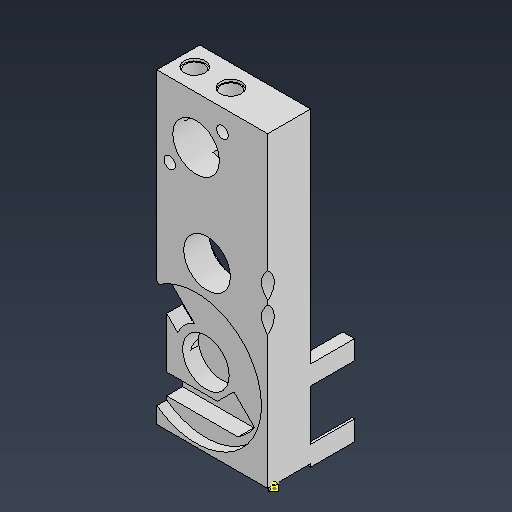
# Autodesk Inventor part: Left_gearbox
Saved by Autodesk Inventor 2026.2 (Build 302298010, 298A)
## iProperties
Created: 2026-04-03
Part Number: Left_gearbox
Material: Generic
Document SubType Name: Modeling
Designer: szymo
Density: 1 g/cm^3
Appearance: Default
Mass: 8.18734 g
Surface Area: 67.5821 cm^2
Volume: 8.18734 cm^3
Author: szymo
Autodesk Inventor part; units mm, degrees
(part 1 of 2)
ref_plane "YZ Plane" through (0, 0, 0) normal (1, 0, 0) x (0, 1, 0)
ref_plane "XZ Plane" through (0, 0, 0) normal (0, 1, 0) x (-1, 0, 0)
ref_plane "XY Plane" through (0, 0, 0) normal (0, 0, 1) x (1, 0, 0)
sketch "Sketch2" plane through (0, 0, 0) normal (0, 0, 1) x (1, 0, 0)
  circle A0 centre (-9.6931, 61.9439) radius 1.0564 construction
  circle A1 centre (-21.0069, 50.6302) radius 1.0564 construction
  circle A2 centre (-15.35, 56.2871) radius 5 projected
  circle A3 centre (-15.35, 56.2871) radius 14 construction
  circle A4 centre (-9.652, 48.0693) radius 1.25 construction
  arc A5 (-9.9568, 54.9375) -> (-10.4245, 56.0319) centre (-14.7581, 53.5328) ccw construction
  arc A6 (-9.5969, 54.944) -> (-9.9568, 54.9375) centre (-9.652, 48.0693) ccw construction
  arc A7 (-9.1694, 56.0547) -> (-9.5969, 54.944) centre (-4.7478, 53.7148) ccw construction
  arc A8 (-8.7521, 56.0185) -> (-9.1694, 56.0547) centre (-9.652, 48.0693) ccw construction
  arc A9 (-8.5222, 54.8508) -> (-8.7521, 56.0185) centre (-13.5106, 54.4751) ccw construction
  arc A10 (-8.1688, 54.7824) -> (-8.5222, 54.8508) centre (-9.652, 48.0693) ccw construction
  arc A11 (-7.5196, 55.7798) -> (-8.1688, 54.7824) centre (-3.6812, 52.5718) ccw construction
  arc A12 (-7.119, 55.6577) -> (-7.5196, 55.7798) centre (-9.652, 48.0693) ccw construction
  arc A13 (-7.1369, 54.4677) -> (-7.119, 55.6577) centre (-12.0944, 55.1373) ccw construction
  arc A14 (-6.8055, 54.3273) -> (-7.1369, 54.4677) centre (-9.652, 48.0693) ccw construction
  arc A15 (-5.9631, 55.168) -> (-6.8055, 54.3273) centre (-2.8755, 51.232) ccw construction
  arc A16 (-5.5966, 54.9652) -> (-5.9631, 55.168) centre (-9.652, 48.0693) ccw construction
  arc A17 (-5.8615, 53.805) -> (-5.5966, 54.9652) centre (-10.5715, 55.4907) ccw construction
  arc A18 (-5.5666, 53.5987) -> (-5.8615, 53.805) centre (-9.652, 48.0693) ccw construction
  arc A19 (-4.5678, 54.2459) -> (-5.5666, 53.5987) centre (-2.366, 49.754) ccw construction
  arc A20 (-4.2515, 53.9714) -> (-4.5678, 54.2459) centre (-9.652, 48.0693) ccw construction
  arc A21 (-4.7519, 52.8916) -> (-4.2515, 53.9714) centre (-9.0084, 55.5197) ccw construction
  arc A22 (-4.5062, 52.6285) -> (-4.7519, 52.8916) centre (-9.652, 48.0693) ccw construction
  arc A23 (-3.3947, 53.0539) -> (-4.5062, 52.6285) centre (-2.175, 48.2023) ccw construction
  arc A24 (-3.1424, 52.7196) -> (-3.3947, 53.0539) centre (-9.652, 48.0693) ccw construction
  arc A25 (-3.8563, 51.7674) -> (-3.1424, 52.7196) centre (-7.4735, 55.2231) ccw construction
  arc A26 (-3.6707, 51.459) -> (-3.8563, 51.7674) centre (-9.652, 48.0693) ccw construction
  arc A27 (-2.4951, 51.644) -> (-3.6707, 51.459) centre (-2.3107, 46.6449) ccw construction
  arc A28 (-2.3178, 51.2646) -> (-2.4951, 51.644) centre (-9.652, 48.0693) ccw construction
  arc A29 (-3.2141, 50.4816) -> (-2.3178, 51.2646) centre (-6.0337, 54.6138) ccw construction
  arc A30 (-3.0967, 50.1413) -> (-3.2141, 50.4816) centre (-9.652, 48.0693) ccw construction
  arc A31 (-1.9082, 50.0779) -> (-3.0967, 50.1413) centre (-2.7673, 45.1497) ccw construction
  arc A32 (-1.8137, 49.6699) -> (-1.9082, 50.0779) centre (-9.652, 48.0693) ccw construction
  arc A33 (-2.8532, 49.0904) -> (-1.8137, 49.6699) centre (-4.7521, 53.7185) ccw construction
  arc A34 (-2.8091, 48.7331) -> (-2.8532, 49.0904) centre (-9.652, 48.0693) ccw construction
  arc A35 (-1.6598, 48.424) -> (-2.8091, 48.7331) centre (-3.5247, 43.7821) ccw construction
  arc A36 (-1.6522, 48.0052) -> (-1.6598, 48.424) centre (-9.652, 48.0693) ccw construction
  arc A37 (-2.7895, 47.6545) -> (-1.6522, 48.0052) centre (-3.6846, 52.5763) ccw construction
  arc A38 (-2.8206, 47.2959) -> (-2.7895, 47.6545) centre (-9.652, 48.0693) ccw construction
  arc A39 (-1.7607, 46.7546) -> (-2.8206, 47.2959) centre (-4.55, 42.6018) ccw construction
  arc A40 (-1.8404, 46.3434) -> (-1.7607, 46.7546) centre (-9.652, 48.0693) ccw construction
  arc A41 (-3.0257, 46.2368) -> (-1.8404, 46.3434) centre (-2.8779, 51.2371) ccw construction
  arc A42 (-3.1307, 45.8925) -> (-3.0257, 46.2368) centre (-9.652, 48.0693) ccw construction
  arc A43 (-2.2065, 45.1426) -> (-3.1307, 45.8925) centre (-5.7982, 41.6605) ccw construction
  arc A44 (-2.3699, 44.757) -> (-2.2065, 45.1426) centre (-9.652, 48.0693) ccw construction
  arc A45 (-3.5515, 44.8991) -> (-2.3699, 44.757) centre (-2.3673, 49.7595) ccw construction
  arc A46 (-3.7258, 44.5842) -> (-3.5515, 44.8991) centre (-9.652, 48.0693) ccw construction
  arc A47 (-2.9777, 43.6586) -> (-3.7258, 44.5842) centre (-7.2149, 40.9993) ccw construction
  arc A48 (-3.2177, 43.3153) -> (-2.9777, 43.6586) centre (-9.652, 48.0693) ccw construction
  arc A49 (-4.3439, 43.7001) -> (-3.2177, 43.3153) centre (-2.1751, 48.208) ccw construction
  arc A50 (-4.5798, 43.4282) -> (-4.3439, 43.7001) centre (-9.652, 48.0693) ccw construction
  arc A51 (-4.0406, 42.3673) -> (-4.5798, 43.4282) centre (-8.7381, 40.6471) ccw construction
  arc A52 (-4.3467, 42.0814) -> (-4.0406, 42.3673) centre (-9.652, 48.0693) ccw construction
  arc A53 (-5.3683, 42.6919) -> (-4.3467, 42.0814) centre (-2.3096, 46.6504) ccw construction
  arc A54 (-5.6556, 42.4751) -> (-5.3683, 42.6919) centre (-9.652, 48.0693) ccw construction
  arc A55 (-5.3487, 41.3252) -> (-5.6556, 42.4751) centre (-10.3012, 40.6193) ccw construction
  arc A56 (-5.7076, 41.1093) -> (-5.3487, 41.3252) centre (-9.652, 48.0693) ccw construction
  arc A57 (-6.5799, 41.9188) -> (-5.7076, 41.1093) centre (-2.7651, 45.1549) ccw construction
  arc A58 (-6.906, 41.7665) -> (-6.5799, 41.9188) centre (-9.652, 48.0693) ccw construction
  arc A59 (-6.8449, 40.5779) -> (-6.906, 41.7665) centre (-11.8359, 40.9171) ccw construction
  arc A60 (-7.2408, 40.4413) -> (-6.8449, 40.5779) centre (-9.652, 48.0693) ccw construction
  arc A61 (-7.9258, 41.4145) -> (-7.2408, 40.4413) centre (-3.5215, 43.7867) ccw construction
  arc A62 (-8.2764, 41.3333) -> (-7.9258, 41.4145) centre (-9.652, 48.0693) ccw construction
  arc A63 (-8.4638, 40.158) -> (-8.2764, 41.3333) centre (-13.2752, 41.5275) ccw construction
  arc A64 (-8.8795, 40.1066) -> (-8.4638, 40.158) centre (-9.652, 48.0693) ccw construction
  arc A65 (-9.3471, 41.201) -> (-8.8795, 40.1066) centre (-4.5458, 42.6057) ccw construction
  arc A66 (-9.707, 41.1945) -> (-9.3471, 41.201) centre (-9.652, 48.0693) ccw construction
  arc A67 (-10.1346, 40.0838) -> (-9.707, 41.1945) centre (-14.5562, 42.4237) ccw construction
  arc A68 (-10.5519, 40.12) -> (-10.1346, 40.0838) centre (-9.652, 48.0693) ccw construction
  arc A69 (-10.7818, 41.2877) -> (-10.5519, 40.12) centre (-5.7934, 41.6635) ccw construction
  arc A70 (-11.1351, 41.3561) -> (-10.7818, 41.2877) centre (-9.652, 48.0693) ccw construction
  arc A71 (-11.7843, 40.3587) -> (-11.1351, 41.3561) centre (-15.6228, 43.5667) ccw construction
  arc A72 (-12.1849, 40.4808) -> (-11.7843, 40.3587) centre (-9.652, 48.0693) ccw construction
  arc A73 (-12.167, 41.6708) -> (-12.1849, 40.4808) centre (-7.2095, 41.0012) ccw construction
  arc A74 (-12.4985, 41.8112) -> (-12.167, 41.6708) centre (-9.652, 48.0693) ccw construction
  arc A75 (-13.3408, 40.9705) -> (-12.4985, 41.8112) centre (-16.4284, 44.9065) ccw construction
  arc A76 (-13.7073, 41.1733) -> (-13.3408, 40.9705) centre (-9.652, 48.0693) ccw construction
  arc A77 (-13.4424, 42.3336) -> (-13.7073, 41.1733) centre (-8.7324, 40.6478) ccw construction
  arc A78 (-13.7374, 42.5398) -> (-13.4424, 42.3336) centre (-9.652, 48.0693) ccw construction
  arc A79 (-14.7361, 41.8926) -> (-13.7374, 42.5398) centre (-16.9379, 46.3845) ccw construction
  arc A80 (-15.0524, 42.1671) -> (-14.7361, 41.8926) centre (-9.652, 48.0693) ccw construction
  arc A81 (-14.5521, 43.247) -> (-15.0524, 42.1671) centre (-10.2955, 40.6188) ccw construction
  arc A82 (-14.7977, 43.51) -> (-14.5521, 43.247) centre (-9.652, 48.0693) ccw construction
  arc A83 (-15.9092, 43.0846) -> (-14.7977, 43.51) centre (-17.129, 47.9362) ccw construction
  arc A84 (-16.1615, 43.4189) -> (-15.9092, 43.0846) centre (-9.652, 48.0693) ccw construction
  arc A85 (-15.4476, 44.3711) -> (-16.1615, 43.4189) centre (-11.8305, 40.9154) ccw construction
  arc A86 (-15.6332, 44.6795) -> (-15.4476, 44.3711) centre (-9.652, 48.0693) ccw construction
  arc A87 (-16.8089, 44.4945) -> (-15.6332, 44.6795) centre (-16.9932, 49.4936) ccw construction
  arc A88 (-16.9861, 44.874) -> (-16.8089, 44.4945) centre (-9.652, 48.0693) ccw construction
  arc A89 (-16.0899, 45.6569) -> (-16.9861, 44.874) centre (-13.2702, 41.5247) ccw construction
  arc A90 (-16.2073, 45.9972) -> (-16.0899, 45.6569) centre (-9.652, 48.0693) ccw construction
  arc A91 (-17.3957, 46.0606) -> (-16.2073, 45.9972) centre (-16.5367, 50.9889) ccw construction
  arc A92 (-17.4902, 46.4687) -> (-17.3957, 46.0606) centre (-9.652, 48.0693) ccw construction
  arc A93 (-16.4507, 47.0482) -> (-17.4902, 46.4687) centre (-14.5519, 42.42) ccw construction
  arc A94 (-16.4948, 47.4054) -> (-16.4507, 47.0482) centre (-9.652, 48.0693) ccw construction
  arc A95 (-17.6441, 47.7145) -> (-16.4948, 47.4054) centre (-15.7792, 52.3565) ccw construction
  arc A96 (-17.6517, 48.1333) -> (-17.6441, 47.7145) centre (-9.652, 48.0693) ccw construction
  arc A97 (-16.5144, 48.484) -> (-17.6517, 48.1333) centre (-15.6193, 43.5622) ccw construction
  arc A98 (-16.4833, 48.8426) -> (-16.5144, 48.484) centre (-9.652, 48.0693) ccw construction
  arc A99 (-17.5432, 49.3839) -> (-16.4833, 48.8426) centre (-14.7539, 53.5367) ccw construction
  arc A100 (-17.4636, 49.7951) -> (-17.5432, 49.3839) centre (-9.652, 48.0693) ccw construction
  arc A101 (-16.2783, 49.9017) -> (-17.4636, 49.7951) centre (-16.426, 44.9014) ccw construction
  arc A102 (-16.1733, 50.246) -> (-16.2783, 49.9017) centre (-9.652, 48.0693) ccw construction
  arc A103 (-17.0974, 50.9959) -> (-16.1733, 50.246) centre (-13.5057, 54.478) ccw construction
  arc A104 (-16.9341, 51.3815) -> (-17.0974, 50.9959) centre (-9.652, 48.0693) ccw construction
  arc A105 (-15.7525, 51.2394) -> (-16.9341, 51.3815) centre (-16.9366, 46.379) ccw construction
  arc A106 (-15.5782, 51.5543) -> (-15.7525, 51.2394) centre (-9.652, 48.0693) ccw construction
  arc A107 (-16.3262, 52.4799) -> (-15.5782, 51.5543) centre (-12.089, 55.1392) ccw construction
  arc A108 (-16.0863, 52.8232) -> (-16.3262, 52.4799) centre (-9.652, 48.0693) ccw construction
  arc A109 (-14.96, 52.4385) -> (-16.0863, 52.8232) centre (-17.1289, 47.9305) ccw construction
  arc A110 (-14.7241, 52.7103) -> (-14.96, 52.4385) centre (-9.652, 48.0693) ccw construction
  arc A111 (-15.2634, 53.7712) -> (-14.7241, 52.7103) centre (-10.5659, 55.4914) ccw construction
  arc A112 (-14.9573, 54.0571) -> (-15.2634, 53.7712) centre (-9.652, 48.0693) ccw construction
  arc A113 (-13.9356, 53.4466) -> (-14.9573, 54.0571) centre (-16.9943, 49.4881) ccw construction
  arc A114 (-13.6483, 53.6634) -> (-13.9356, 53.4466) centre (-9.652, 48.0693) ccw construction
  arc A115 (-13.9552, 54.8133) -> (-13.6483, 53.6634) centre (-9.0028, 55.5192) ccw construction
  arc A116 (-13.5964, 55.0293) -> (-13.9552, 54.8133) centre (-9.652, 48.0693) ccw construction
  arc A117 (-12.724, 54.2197) -> (-13.5964, 55.0293) centre (-16.5389, 50.9836) ccw construction
  arc A118 (-12.3979, 54.3721) -> (-12.724, 54.2197) centre (-9.652, 48.0693) ccw construction
  arc A119 (-12.459, 55.5606) -> (-12.3979, 54.3721) centre (-7.468, 55.2214) ccw construction
  arc A120 (-12.0631, 55.6973) -> (-12.459, 55.5606) centre (-9.652, 48.0693) ccw construction
  arc A121 (-11.3781, 54.724) -> (-12.0631, 55.6973) centre (-15.7825, 52.3518) ccw construction
  arc A122 (-11.0275, 54.8052) -> (-11.3781, 54.724) centre (-9.652, 48.0693) ccw construction
  arc A123 (-10.8402, 55.9805) -> (-11.0275, 54.8052) centre (-6.0287, 54.6111) ccw construction
  arc A124 (-10.4245, 56.0319) -> (-10.8402, 55.9805) centre (-9.652, 48.0693) ccw construction
  circle A125 centre (-13, 35.9222) radius 5 projected
  arc A126 (-10.4838, 26.6578) -> (-10.4239, 28.0847) centre (-16.409, 27.6212) ccw construction
  arc A127 (-10.4239, 28.0847) -> (-10.0173, 28.2303) centre (-13, 35.9222) ccw construction
  arc A128 (-10.0173, 28.2303) -> (-9.0655, 27.1655) centre (-5.0975, 31.6701) ccw construction
  arc A129 (-9.0655, 27.1655) -> (-8.6126, 27.3834) centre (-13, 35.9222) ccw construction
  arc A130 (-8.6126, 27.3834) -> (-8.8507, 28.7916) centre (-14.6087, 27.0938) ccw construction
  arc A131 (-8.8507, 28.7916) -> (-8.4832, 29.0185) centre (-13, 35.9222) ccw construction
  arc A132 (-8.4832, 29.0185) -> (-7.3309, 28.1749) centre (-4.3862, 33.4061) ccw construction
  arc A133 (-7.3309, 28.1749) -> (-6.9332, 28.4822) centre (-13, 35.9222) ccw construction
  arc A134 (-6.9332, 28.4822) -> (-7.4588, 29.8101) centre (-12.738, 26.9522) ccw construction
  arc A135 (-7.4588, 29.8101) -> (-7.1466, 30.1085) centre (-13, 35.9222) ccw construction
  arc A136 (-7.1466, 30.1085) -> (-5.844, 29.5229) centre (-4.0513, 35.252) ccw construction
  arc A137 (-5.844, 29.5229) -> (-5.5189, 29.9062) centre (-13, 35.9222) ccw construction
  arc A138 (-5.5189, 29.9062) -> (-6.3091, 31.0957) centre (-10.8787, 27.2027) ccw construction
  arc A139 (-6.3091, 31.0957) -> (-6.0657, 31.4525) centre (-13, 35.9222) ccw construction
  arc A140 (-6.0657, 31.4525) -> (-4.6699, 31.1505) centre (-4.1075, 37.1272) ccw construction
  arc A141 (-4.6699, 31.1505) -> (-4.4316, 31.593) centre (-13, 35.9222) ccw construction
  arc A142 (-4.4316, 31.593) -> (-5.4519, 32.5923) centre (-9.1122, 27.8343) ccw construction
  arc A143 (-5.4519, 32.5923) -> (-5.2879, 32.9919) centre (-13, 35.9222) ccw construction
  arc A144 (-5.2879, 32.9919) -> (-3.8598, 32.9867) centre (-4.5523, 38.9497) ccw construction
  arc A145 (-3.8598, 32.9867) -> (-3.7187, 33.4691) centre (-13, 35.9222) ccw construction
  arc A146 (-3.7187, 33.4691) -> (-4.9245, 34.2344) centre (-7.5156, 28.8194) ccw construction
  arc A147 (-4.9245, 34.2344) -> (-4.8472, 34.6594) centre (-13, 35.9222) ccw construction
  arc A148 (-4.8472, 34.6594) -> (-3.4492, 34.9512) centre (-5.3664, 40.6399) ccw construction
  arc A149 (-3.4492, 34.9512) -> (-3.4115, 35.4524) centre (-13, 35.9222) ccw construction
  arc A150 (-3.4115, 35.4524) -> (-4.75, 35.9503) centre (-6.1587, 30.1148) ccw construction
  arc A151 (-4.75, 35.9503) -> (-4.7628, 36.382) centre (-13, 35.9222) ccw construction
  arc A152 (-4.7628, 36.382) -> (-3.4561, 36.9582) centre (-6.514, 42.124) ccw construction
  arc A153 (-3.4561, 36.9582) -> (-3.5234, 37.4562) centre (-13, 35.9222) ccw construction
  arc A154 (-3.5234, 37.4562) -> (-4.9362, 37.6649) centre (-5.1008, 31.6641) ccw construction
  arc A155 (-4.9362, 37.6649) -> (-5.0384, 38.0846) centre (-13, 35.9222) ccw construction
  arc A156 (-5.0384, 38.0846) -> (-3.88, 38.9198) centre (-7.9452, 43.3369) ccw construction
  arc A157 (-3.88, 38.9198) -> (-4.0494, 39.393) centre (-13, 35.9222) ccw construction
  arc A158 (-4.0494, 39.393) -> (-5.4747, 39.3034) centre (-4.3881, 33.3995) ccw construction
  arc A159 (-5.4747, 39.3034) -> (-5.662, 39.6926) centre (-13, 35.9222) ccw construction
  arc A160 (-5.662, 39.6926) -> (-4.7025, 40.7505) centre (-9.5973, 44.2259) ccw construction
  arc A161 (-4.7025, 40.7505) -> (-4.9666, 41.1781) centre (-13, 35.9222) ccw construction
  arc A162 (-4.9666, 41.1781) -> (-6.3422, 40.7941) centre (-4.0518, 35.2452) ccw construction
  arc A163 (-6.3422, 40.7941) -> (-6.6063, 41.1359) centre (-13, 35.9222) ccw construction
  arc A164 (-6.6063, 41.1359) -> (-5.8877, 42.3701) centre (-11.398, 44.7519) ccw construction
  arc A165 (-5.8877, 42.3701) -> (-6.2349, 42.7335) centre (-13, 35.9222) ccw construction
  arc A166 (-6.2349, 42.7335) -> (-7.5006, 42.0719) centre (-4.1066, 37.1204) ccw construction
  arc A167 (-7.5006, 42.0719) -> (-7.83, 42.3513) centre (-13, 35.9222) ccw construction
  arc A168 (-7.83, 42.3513) -> (-7.3837, 43.7079) centre (-13.2688, 44.892) ccw construction
  arc A169 (-7.3837, 43.7079) -> (-7.7989, 43.9912) centre (-13, 35.9222) ccw construction
  arc A170 (-7.7989, 43.9912) -> (-8.8993, 43.0809) centre (-4.55, 38.9433) ccw construction
  arc A171 (-8.8993, 43.0809) -> (-9.2796, 43.2857) centre (-13, 35.9222) ccw construction
  arc A172 (-9.2796, 43.2857) -> (-9.1252, 44.7055) centre (-15.1279, 44.6401) ccw construction
  arc A173 (-9.1252, 44.7055) -> (-9.5902, 44.8962) centre (-13, 35.9222) ccw construction
  arc A174 (-9.5902, 44.8962) -> (-10.4773, 43.7771) centre (-5.3628, 40.6341) ccw construction
  arc A175 (-10.4773, 43.7771) -> (-10.8919, 43.8983) centre (-13, 35.9222) ccw construction
  arc A176 (-10.8919, 43.8983) -> (-11.036, 45.3192) centre (-16.8939, 44.0072) ccw construction
  arc A177 (-11.036, 45.3192) -> (-11.5305, 45.4091) centre (-13, 35.9222) ccw construction
  arc A178 (-11.5305, 45.4091) -> (-12.1656, 44.1299) centre (-6.5093, 42.119) ccw construction
  arc A179 (-12.1656, 44.1299) -> (-12.5963, 44.1623) centre (-13, 35.9222) ccw construction
  arc A180 (-12.5963, 44.1623) -> (-13.0327, 45.5222) centre (-18.4898, 43.0209) ccw construction
  arc A181 (-13.0327, 45.5222) -> (-13.535, 45.5073) centre (-13, 35.9222) ccw construction
  arc A182 (-13.535, 45.5073) -> (-13.8903, 44.124) centre (-7.9396, 43.3331) ccw construction
  arc A183 (-13.8903, 44.124) -> (-14.3183, 44.0662) centre (-13, 35.9222) ccw construction
  arc A184 (-14.3183, 44.0662) -> (-15.0279, 45.3056) centre (-19.8457, 41.7244) ccw construction
  arc A185 (-15.0279, 45.3056) -> (-15.5162, 45.1866) centre (-13, 35.9222) ccw construction
  arc A186 (-15.5162, 45.1866) -> (-15.5761, 43.7597) centre (-9.591, 44.2233) ccw construction
  arc A187 (-15.5761, 43.7597) -> (-15.9827, 43.6141) centre (-13, 35.9222) ccw construction
  arc A188 (-15.9827, 43.6141) -> (-16.9345, 44.6789) centre (-20.9025, 40.1743) ccw construction
  arc A189 (-16.9345, 44.6789) -> (-17.3874, 44.461) centre (-13, 35.9222) ccw construction
  arc A190 (-17.3874, 44.461) -> (-17.1493, 43.0528) centre (-11.3913, 44.7507) ccw construction
  arc A191 (-17.1493, 43.0528) -> (-17.5168, 42.8259) centre (-13, 35.9222) ccw construction
  arc A192 (-17.5168, 42.8259) -> (-18.6691, 43.6695) centre (-21.6138, 38.4383) ccw construction
  arc A193 (-18.6691, 43.6695) -> (-19.0668, 43.3622) centre (-13, 35.9222) ccw construction
  arc A194 (-19.0668, 43.3622) -> (-18.5412, 42.0343) centre (-13.262, 44.8922) ccw construction
  arc A195 (-18.5412, 42.0343) -> (-18.8534, 41.736) centre (-13, 35.9222) ccw construction
  arc A196 (-18.8534, 41.736) -> (-20.156, 42.3216) centre (-21.9487, 36.5924) ccw construction
  arc A197 (-20.156, 42.3216) -> (-20.4811, 41.9383) centre (-13, 35.9222) ccw construction
  arc A198 (-20.4811, 41.9383) -> (-19.6909, 40.7487) centre (-15.1213, 44.6417) ccw construction
  arc A199 (-19.6909, 40.7487) -> (-19.9343, 40.3919) centre (-13, 35.9222) ccw construction
  arc A200 (-19.9343, 40.3919) -> (-21.3301, 40.6939) centre (-21.8925, 34.7172) ccw construction
  arc A201 (-21.3301, 40.6939) -> (-21.5684, 40.2514) centre (-13, 35.9222) ccw construction
  arc A202 (-21.5684, 40.2514) -> (-20.5481, 39.2521) centre (-16.8878, 44.0101) ccw construction
  arc A203 (-20.5481, 39.2521) -> (-20.7121, 38.8525) centre (-13, 35.9222) ccw construction
  arc A204 (-20.7121, 38.8525) -> (-22.1402, 38.8577) centre (-21.4477, 32.8947) ccw construction
  arc A205 (-22.1402, 38.8577) -> (-22.2813, 38.3753) centre (-13, 35.9222) ccw construction
  arc A206 (-22.2813, 38.3753) -> (-21.0755, 37.61) centre (-18.4844, 43.0251) ccw construction
  arc A207 (-21.0755, 37.61) -> (-21.1528, 37.1851) centre (-13, 35.9222) ccw construction
  arc A208 (-21.1528, 37.1851) -> (-22.5508, 36.8932) centre (-20.6336, 31.2045) ccw construction
  arc A209 (-22.5508, 36.8932) -> (-22.5885, 36.392) centre (-13, 35.9222) ccw construction
  arc A210 (-22.5885, 36.392) -> (-21.25, 35.8941) centre (-19.8413, 41.7296) ccw construction
  arc A211 (-21.25, 35.8941) -> (-21.2372, 35.4624) centre (-13, 35.9222) ccw construction
  arc A212 (-21.2372, 35.4624) -> (-22.5439, 34.8863) centre (-19.486, 29.7205) ccw construction
  arc A213 (-22.5439, 34.8863) -> (-22.4766, 34.3882) centre (-13, 35.9222) ccw construction
  arc A214 (-22.4766, 34.3882) -> (-21.0638, 34.1795) centre (-20.8992, 40.1803) ccw construction
  arc A215 (-21.0638, 34.1795) -> (-20.9616, 33.7599) centre (-13, 35.9222) ccw construction
  arc A216 (-20.9616, 33.7599) -> (-22.12, 32.9246) centre (-18.0548, 28.5075) ccw construction
  arc A217 (-22.12, 32.9246) -> (-21.9506, 32.4514) centre (-13, 35.9222) ccw construction
  arc A218 (-21.9506, 32.4514) -> (-20.5253, 32.541) centre (-21.6119, 38.4449) ccw construction
  arc A219 (-20.5253, 32.541) -> (-20.338, 32.1518) centre (-13, 35.9222) ccw construction
  arc A220 (-20.338, 32.1518) -> (-21.2975, 31.0939) centre (-16.4027, 27.6186) ccw construction
  arc A221 (-21.2975, 31.0939) -> (-21.0334, 30.6663) centre (-13, 35.9222) ccw construction
  arc A222 (-21.0334, 30.6663) -> (-19.6578, 31.0503) centre (-21.9482, 36.5992) ccw construction
  arc A223 (-19.6578, 31.0503) -> (-19.3937, 30.7085) centre (-13, 35.9222) ccw construction
  arc A224 (-19.3937, 30.7085) -> (-20.1123, 29.4743) centre (-14.602, 27.0926) ccw construction
  arc A225 (-20.1123, 29.4743) -> (-19.7651, 29.1109) centre (-13, 35.9222) ccw construction
  arc A226 (-19.7651, 29.1109) -> (-18.4994, 29.7725) centre (-21.8934, 34.724) ccw construction
  arc A227 (-18.4994, 29.7725) -> (-18.17, 29.4931) centre (-13, 35.9222) ccw construction
  arc A228 (-18.17, 29.4931) -> (-18.6163, 28.1365) centre (-12.7312, 26.9524) ccw construction
  arc A229 (-18.6163, 28.1365) -> (-18.2011, 27.8532) centre (-13, 35.9222) ccw construction
  arc A230 (-18.2011, 27.8532) -> (-17.1007, 28.7635) centre (-21.45, 32.9011) ccw construction
  arc A231 (-17.1007, 28.7635) -> (-16.7204, 28.5587) centre (-13, 35.9222) ccw construction
  arc A232 (-16.7204, 28.5587) -> (-16.8748, 27.1389) centre (-10.8721, 27.2043) ccw construction
  arc A233 (-16.8748, 27.1389) -> (-16.4098, 26.9482) centre (-13, 35.9222) ccw construction
  arc A234 (-16.4098, 26.9482) -> (-15.5227, 28.0674) centre (-20.6372, 31.2103) ccw construction
  arc A235 (-15.5227, 28.0674) -> (-15.1081, 27.9461) centre (-13, 35.9222) ccw construction
  arc A236 (-15.1081, 27.9461) -> (-14.964, 26.5253) centre (-9.1061, 27.8373) ccw construction
  arc A237 (-14.964, 26.5253) -> (-14.4695, 26.4353) centre (-13, 35.9222) ccw construction
  arc A238 (-14.4695, 26.4353) -> (-13.8344, 27.7145) centre (-19.4907, 29.7254) ccw construction
  arc A239 (-13.8344, 27.7145) -> (-13.4037, 27.6821) centre (-13, 35.9222) ccw construction
  arc A240 (-13.4037, 27.6821) -> (-12.9673, 26.3223) centre (-7.5102, 28.8235) ccw construction
  arc A241 (-12.9673, 26.3223) -> (-12.465, 26.3371) centre (-13, 35.9222) ccw construction
  arc A242 (-12.465, 26.3371) -> (-12.1097, 27.7204) centre (-18.0604, 28.5113) ccw construction
  arc A243 (-12.1097, 27.7204) -> (-11.6817, 27.7782) centre (-13, 35.9222) ccw construction
  arc A244 (-11.6817, 27.7782) -> (-10.9721, 26.5388) centre (-6.1543, 30.12) ccw construction
  arc A245 (-10.9721, 26.5388) -> (-10.4838, 26.6578) centre (-13, 35.9222) ccw construction
  line L0 (0, 0.65) -> (-23.75, 0.65)
  line L1 (-23.75, 0.65) -> (-23.75, 66.4871)
  line L2 (-23.75, 66.4871) -> (0, 66.4871)
  line L3 (0, 66.4871) -> (0, 0.65)
  circle A246 centre (-13, 35.9222) radius 9.6
  circle A247 centre (-9.652, 48.0693) radius 8
  line L4 (-15.35, 66.4871) -> (-15.35, 56.2871) construction
  circle A248 centre (-15.35, 56.2871) radius 14.7 construction
  circle A249 centre (-15.35, 15.35) radius 14.7 construction
  line L5 (-15.35, 66.4871) -> (-15.35, 70.9871) construction
  circle A250 centre (-9.652, 48.0693) radius 8.4
  circle A251 centre (-13, 35.9222) radius 10
  line L6 (-21.3604, 17.8249) -> (-25.778, 22.2425)
  arc A252 (-23.75, 27.2855) -> (-25.778, 22.2425) centre (-13.4441, 20.2118) ccw
  line L7 (-23.75, 27.2855) -> (-17.8249, 21.3604)
  arc A253 (-17.8249, 21.3604) -> (-21.3604, 17.8249) centre (-15.35, 15.35) ccw construction
  line L8 (-9.3396, 12.8751) -> (-4.922, 8.4575)
  arc A254 (-8.4575, 4.922) -> (-4.922, 8.4575) centre (-15.35, 15.35) ccw
  line L9 (-8.4575, 4.922) -> (-12.8751, 9.3396)
  arc A255 (-12.8751, 9.3396) -> (-9.3396, 12.8751) centre (-15.35, 15.35) ccw construction
  line L10 (-17.8249, 21.3604) -> (-21.3604, 17.8249)
  line L11 (-9.3396, 12.8751) -> (-12.8751, 9.3396)
  line L12 (-12.8751, 9.3396) -> (-23.75, 9.3396)
  line L13 (-8.4575, 4.922) -> (-23.75, 4.922)
  line L14 (-21.3604, 17.8249) -> (-25.778, 22.2425)
  arc A256 (-23.75, 27.2855) -> (-25.778, 22.2425) centre (-13.4441, 20.2118) ccw
  line L15 (-23.75, 27.2855) -> (-17.8249, 21.3604)
  arc A257 (-17.8249, 21.3604) -> (-21.3604, 17.8249) centre (-15.35, 15.35) ccw
  arc A258 (-8.4575, 4.922) -> (-4.922, 8.4575) centre (-15.35, 15.35) ccw
  line L16 (-4.922, 8.4575) -> (-9.3396, 12.8751)
  arc A259 (-12.8751, 9.3396) -> (-9.3396, 12.8751) centre (-15.35, 15.35) ccw
  line L17 (-12.8751, 9.3396) -> (-8.4575, 4.922)
  line L18 (-19.4855, 21.6068) -> (-22.3516, 24.4729) projected
  arc A260 (-22.3516, 24.4729) -> (-24.4729, 22.3516) centre (-15.35, 15.35) ccw projected
  line L19 (-24.4729, 22.3516) -> (-21.6068, 19.4855) projected
  arc A261 (-19.4855, 21.6068) -> (-21.6068, 19.4855) centre (-15.35, 15.35) ccw projected
  arc A262 (-8.3484, 6.2271) -> (-6.2271, 8.3484) centre (-15.35, 15.35) ccw projected
  line L20 (-6.2271, 8.3484) -> (-9.0932, 11.2145) projected
  arc A263 (-11.2145, 9.0932) -> (-9.0932, 11.2145) centre (-15.35, 15.35) ccw projected
  line L21 (-11.2145, 9.0932) -> (-8.3484, 6.2271) projected
  circle A264 centre (-15.35, 15.35) radius 5 projected
  circle A265 centre (-15.35, 15.35) radius 14 projected
  circle A266 centre (-9.652, 48.0693) radius 1.25 construction
  arc A267 (-10.7292, 45.4307) -> (-10.7184, 44.0069) centre (-7.0884, 44.7465) ccw construction
  arc A268 (-11.0644, 45.5939) -> (-10.7292, 45.4307) centre (-9.652, 48.0693) ccw construction
  arc A269 (-12.1918, 44.7242) -> (-11.0644, 45.5939) centre (-13.8486, 48.0376) ccw construction
  arc A270 (-12.6067, 45.0843) -> (-12.1918, 44.7242) centre (-9.652, 48.0693) ccw construction
  arc A271 (-11.9042, 46.3228) -> (-12.6067, 45.0843) centre (-9.0932, 43.9099) ccw construction
  arc A272 (-12.1129, 46.6317) -> (-11.9042, 46.3228) centre (-9.652, 48.0693) ccw construction
  arc A273 (-13.524, 46.4423) -> (-12.1129, 46.6317) centre (-13.3022, 50.1402) ccw construction
  arc A274 (-13.7033, 46.9616) -> (-13.524, 46.4423) centre (-9.652, 48.0693) ccw construction
  arc A275 (-12.4757, 47.6829) -> (-13.7033, 46.9616) centre (-11.2478, 44.1877) ccw construction
  arc A276 (-12.5019, 48.0548) -> (-12.4757, 47.6829) centre (-9.652, 48.0693) ccw construction
  arc A277 (-13.8188, 48.5963) -> (-12.5019, 48.0548) centre (-11.7777, 51.6878) ccw construction
  arc A278 (-13.7143, 49.1357) -> (-13.8188, 48.5963) centre (-9.652, 48.0693) ccw construction
  arc A279 (-12.2905, 49.1465) -> (-13.7143, 49.1357) centre (-12.9747, 45.5057) ccw construction
  arc A280 (-12.1274, 49.4817) -> (-12.2905, 49.1465) centre (-9.652, 48.0693) ccw construction
  arc A281 (-12.997, 50.6091) -> (-12.1274, 49.4817) centre (-9.6836, 52.2659) ccw construction
  arc A282 (-12.6369, 51.024) -> (-12.997, 50.6091) centre (-9.652, 48.0693) ccw construction
  arc A283 (-11.3984, 50.3215) -> (-12.6369, 51.024) centre (-13.8114, 47.5105) ccw construction
  arc A284 (-11.0895, 50.5302) -> (-11.3984, 50.3215) centre (-9.652, 48.0693) ccw construction
  arc A285 (-11.279, 51.9413) -> (-11.0895, 50.5302) centre (-7.5811, 51.7195) ccw construction
  arc A286 (-10.7596, 52.1206) -> (-11.279, 51.9413) centre (-9.652, 48.0693) ccw construction
  arc A287 (-10.0383, 50.8929) -> (-10.7596, 52.1206) centre (-13.5335, 49.6651) ccw construction
  arc A288 (-9.6665, 50.9192) -> (-10.0383, 50.8929) centre (-9.652, 48.0693) ccw construction
  arc A289 (-9.1249, 52.2361) -> (-9.6665, 50.9192) centre (-6.0334, 50.195) ccw construction
  arc A290 (-8.5856, 52.1316) -> (-9.1249, 52.2361) centre (-9.652, 48.0693) ccw construction
  arc A291 (-8.5747, 50.7078) -> (-8.5856, 52.1316) centre (-12.2156, 51.392) ccw construction
  arc A292 (-8.2395, 50.5446) -> (-8.5747, 50.7078) centre (-9.652, 48.0693) ccw construction
  arc A293 (-7.1122, 51.4143) -> (-8.2395, 50.5446) centre (-5.4553, 48.1009) ccw construction
  arc A294 (-6.6973, 51.0542) -> (-7.1122, 51.4143) centre (-9.652, 48.0693) ccw construction
  arc A295 (-7.3998, 49.8157) -> (-6.6973, 51.0542) centre (-10.2107, 52.2286) ccw construction
  arc A296 (-7.1911, 49.5068) -> (-7.3998, 49.8157) centre (-9.652, 48.0693) ccw construction
  arc A297 (-5.7799, 49.6962) -> (-7.1911, 49.5068) centre (-6.0018, 45.9983) ccw construction
  arc A298 (-5.6007, 49.1769) -> (-5.7799, 49.6962) centre (-9.652, 48.0693) ccw construction
  arc A299 (-6.8283, 48.4556) -> (-5.6007, 49.1769) centre (-8.0562, 51.9508) ccw construction
  arc A300 (-6.802, 48.0838) -> (-6.8283, 48.4556) centre (-9.652, 48.0693) ccw construction
  arc A301 (-5.4852, 47.5422) -> (-6.802, 48.0838) centre (-7.5263, 44.4507) ccw construction
  arc A302 (-5.5896, 47.0029) -> (-5.4852, 47.5422) centre (-9.652, 48.0693) ccw construction
  arc A303 (-7.0134, 46.992) -> (-5.5896, 47.0029) centre (-6.3292, 50.6328) ccw construction
  arc A304 (-7.1766, 46.6568) -> (-7.0134, 46.992) centre (-9.652, 48.0693) ccw construction
  arc A305 (-6.3069, 45.5294) -> (-7.1766, 46.6568) centre (-9.6203, 43.8726) ccw construction
  arc A306 (-6.6671, 45.1146) -> (-6.3069, 45.5294) centre (-9.652, 48.0693) ccw construction
  arc A307 (-7.9055, 45.8171) -> (-6.6671, 45.1146) centre (-5.4926, 48.628) ccw construction
  arc A308 (-8.2144, 45.6084) -> (-7.9055, 45.8171) centre (-9.652, 48.0693) ccw construction
  arc A309 (-8.025, 44.1972) -> (-8.2144, 45.6084) centre (-11.7229, 44.4191) ccw construction
  arc A310 (-8.5443, 44.018) -> (-8.025, 44.1972) centre (-9.652, 48.0693) ccw construction
  arc A311 (-9.2656, 45.2456) -> (-8.5443, 44.018) centre (-5.7705, 46.4734) ccw construction
  arc A312 (-9.6375, 45.2193) -> (-9.2656, 45.2456) centre (-9.652, 48.0693) ccw construction
  arc A313 (-10.179, 43.9025) -> (-9.6375, 45.2193) centre (-13.2705, 45.9435) ccw construction
  arc A314 (-10.7184, 44.0069) -> (-10.179, 43.9025) centre (-9.652, 48.0693) ccw construction
  circle A315 centre (-9.652, 48.0693) radius 4.2 construction
  circle A316 centre (-9.652, 48.0693) radius 4.6
  point P0 (-23.75, 5.9421)
  point P1 (-23.75, 21.0885)
  point P2 (-16.9043, 44.6924)
  point P3 (-16.868, 51.5231)
  point P4 (-10.3562, 56.0382)
  point P5 (-5.1538, 41.4537)
  point P6 (-17.4267, 44.8891)
  point P7 (-17.2457, 51.6604)
  point P8 (-10.3523, 56.44)
  point P9 (-4.6044, 41.3549)
  point P10 (-23.75, 24.7122)
  point P11 (-3.7958, 23.2888)
  point P12 (-4.9302, 41.122)
  point P13 (-9.6896, 39.6693)
  point P14 (-13.9232, 40.8362)
  point P15 (-17.2663, 44.5221)
  point P16 (-23.75, 25.5904)
  point P17 (-23.75, 20.2145)
  point P18 (-17.0641, 45.0591)
  point P19 (-4.8287, 41.6868)
  point P20 (-23.2, 22.4097)
  point P21 (-23.75, 25.5904)
  point P22 (-23.75, 4.15)
  point P23 (-23.75, 26.55)
  point P24 (-23.75, 20.2145)
  point P25 (-23.3226, 26.8581)
  dimension "d2" = 4.5
  dimension "d14" = 0.4
  dimension "d15" = 0.4
  dimension "d37" = 0.75
  dimension "d121" = 1
  dimension "d122" = 1
  dimension "d123" = 1
  dimension "d124" = 1
  dimension "d125" = 1
  dimension "d126" = 1
  dimension "d127" = 0.4
  dimension "d145" = 0
  constraints: 36 end point, 16 point on circle, 12 centre point, 7 point on line, 6 perpendicular, 3 coincident, 3 concentric, 2 vertical, 1 horizontal, 1 parallel, 1 vertical alignment, 8 other
  measures "d2" distance of L4.start L5.end
  measures "d15" radial gap between concentric circles of A246 A251
  measures "d37" distance edge to line of A251 L1
  measures "d121" distance between parallel lines of L6 L19
  measures "d122" distance between parallel lines of L7 L18
  measures "d123" radial gap between concentric circles of A259 A263
  measures "d124" distance between parallel lines of L8 L20
  measures "d125" distance between parallel lines of L17 L21
  measures "d126" radial gap between concentric circles of A261 A257
  measures "d145" distance edge to line of A249 L0
ref_plane "Work Plane3" through (-33.4195, -4.4195, -0.6) normal (0, 0, -1) x (-0.5, 0.8660254, 0)
ref_plane "Work Plane4" through (-33.7893, 35.5042, 0.6) normal (0, 0, -1) x (-0.5735764, 0.819152, 0)
ref_plane "Work Plane7" through (-34.0123, 35.7835, 2.1) normal (0, 0, -1) x (-0.6427876, 0.7660444, 0)
extrude "Extrusion3" add sketch "Sketch2" along normal up to surface (2.1 mm away) contours A2 A250 A251 A247 | A2 A250 A251 A265 L7 L1 L2 L3 L0 | A247 A251 A316 A2 | A2 A247 A251 A250 | A251 A247 A246 A250 | A250 A246 A265 A251 | A251 A265 A246 A250 | A250 A246 A247 A251 | A251 A316 A246 A247 | A247 A246 A316 A251 | A250 A125 A246 A265 | A246 A247 A125 A250 | A250 A125 A247 A246 | A246 A316 A247 A125
extrude "Extrusion4" add sketch "Sketch2" against normal blind 1 contours A2 A250 A251 A247 | A2 A250 A251 A265 L7 L1 L2 L3 L0 | A247 A251 A316 A2 | A2 A247 A251 A250 | A251 A247 A246 A250 | A250 A246 A265 A251 | A251 A265 A246 A250 | A250 A246 A247 A251 | A251 A316 A246 A247 | A247 A246 A316 A251 | A250 A125 A246 A265 | A246 A247 A125 A250 | A265 A246 A251 | A251 A265 L1 L13 A254 L8 L11 L12 L6 L10 L7 | A250 A125 A247 A246 | A246 A316 A247 A125 | A265 A246
extrude "Extrusion5" add sketch "Sketch2" against normal blind 3.4 contours A2 A250 A251 A247 | A2 A250 A251 A265 L7 L1 L2 L3 L0 | A247 A251 A316 A2 | A2 A247 A251 A250 | A251 A247 A246 A250 | A250 A246 A265 A251 | A251 A265 A246 A250 | A250 A246 A247 A251 | A251 A316 A246 A247 | A247 A246 A316 A251 | A250 A125 A246 A265 | A246 A247 A125 A250 | A265 A246 A251 | A251 A265 L1 L13 A254 L8 L11 L12 L6 L10 L7 | A250 A125 A247 A246 | A246 A316 A247 A125 | A265 A246 | L10 A257
ref_plane "Work Plane5" through (0, 0, -3.4) normal (0, 0, -1) x (-1, 0, 0)